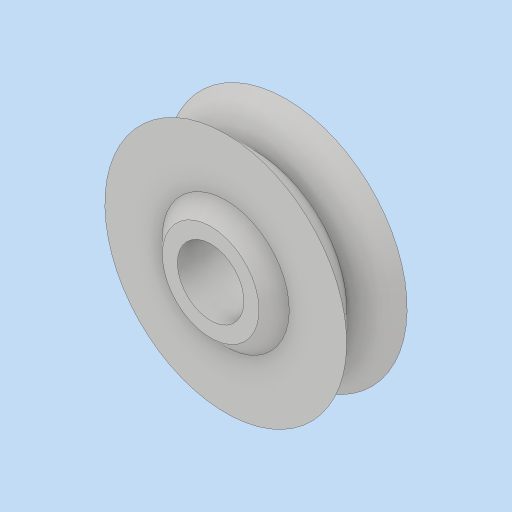
# Autodesk Inventor part: wheel-4-12
Saved by Autodesk Inventor 2024 (Build 280153000, 153)
## iProperties
Created: 2022-10-19
Part Number: wheel-4-12
Material: Generic
Document SubType Name: Modeling
Designer: Karbosch
Mass: 0.61525 g
Surface Area: 7.22712 cm^2
Volume: 0.61525 cm^3
Density: 1 g/cm^3
Appearance: Default
Author: Karbosch
Autodesk Inventor part; units mm, degrees
ref_plane "YZ Plane" through (0, 0, 0) normal (1, 0, 0) x (0, 1, 0)
ref_plane "XZ Plane" through (0, 0, 0) normal (0, 1, 0) x (-1, 0, 0)
ref_plane "XY Plane" through (0, 0, 0) normal (0, 0, 1) x (1, 0, 0)
sketch "Sketch90" plane through (0, 0, 0) normal (0, 0, 1) x (1, 0, 0)
  circle A0 centre (0, 0) radius 2.2
  circle A1 centre (0, 0) radius 6
  dimension "d450" = 4.4
  dimension "d451" = 12
  constraints: 2 centre point, 2 coincident
  measures "d450" diameter of A0
  measures "d451" diameter of A1
extrude "Extrusion69" add sketch "Sketch90" along normal blind 4
sketch "Sketch91" plane through (0, 0, 0) normal (1, 0, 0) x (0, 1, 0)
  line L0 (6, 0) -> (6, 4) projected
  line L1 (6, 4) -> (8, 4)
  line L2 (6, 0) -> (8, 0)
  line L3 (8, 4) -> (6, 2)
  line L4 (8, 0) -> (6, 2)
  line L5 (0, 0) -> (0, -8)
  line L6 (2.2, 0) -> (-2.2, 0) projected
  line L7 (-6, 0) -> (6, 0) projected
  line L8 (-2.2, 4) -> (2.2, 4) projected
  line L9 (6, 4) -> (-6, 4) projected
  line L10 (-2.2, 4) -> (2.2, 4) projected
  line L11 (2.2, 0) -> (-2.2, 0) projected
  line L12 (2.2, 0) -> (-2.2, 0) projected
  line L13 (2.2, 0) -> (2.2, 4) projected
  line L14 (2.2, 0) -> (4.2, 0)
  line L15 (4.2, 0) -> (4.2, 0)
  line L16 (3.2, -1) -> (2.2, -1)
  line L17 (2.2, -1) -> (2.2, 0)
  line L18 (-2.2, 4) -> (2.2, 4) projected
  line L19 (2.2, 4) -> (4.2, 4)
  line L20 (4.2, 4) -> (4.2, 4)
  line L21 (3.2, 5) -> (2.2, 5)
  line L22 (2.2, 5) -> (2.2, 4)
  line L23 (4.2, 0) -> (3.2, -1)
  line L24 (4.2, 4) -> (3.2, 5)
  point P0 (4.2, -1)
  point P1 (4.2, 5)
  dimension "d454" = 2
  dimension "d456" = 2
  dimension "d457" = 1
  dimension "d458" = 1
  dimension "d459" = 1
  dimension "d460" = 1
  dimension "d461" = 1
  dimension "d462" = 1
  constraints: 30 end point, 6 parallel, 5 point on line, 3 horizontal, 2 perpendicular, 1 midpoint, 1 vertical
  measures "d454" distance of L0.end L1.end
  measures "d456" distance of point (4.2, -1) L16.end
  measures "d457" distance of L14.end point (4.2, -1)
  measures "d458" distance of point (4.2, 5) L19.end
  measures "d459" distance of L15.end point (4.2, -1)
  measures "d460" distance of L16.start point (4.2, -1)
  measures "d461" distance of L20.end point (4.2, 5)
  measures "d462" distance of L21.start point (4.2, 5)
revolve "Revolution9" add sketch "Sketch91" angle 360 about axis through (0, 0, 0) along (0, 0, -1) contours L0 L4 L2 | L0 L1 L3 | L23 L16 L17 L7 | L9 L22 L21 L24
body "Solid7"
